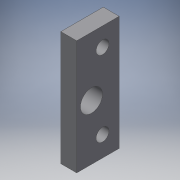
# Autodesk Inventor part: TrayPanelL
Saved by Autodesk Inventor 2017 (Build 210142000, 142)
## iProperties
Created: 2019-06-29
Part Number: TrayPanelL
Material: Generic
Document SubType Name: Modeling
Designer: DDeGo
Density: 1 g/cm^3
Appearance: Default
Author: DDeGo
Autodesk Inventor part; units mm, degrees
ref_plane "YZ Plane" through (0, 0, 0) normal (1, 0, 0) x (0, 1, 0)
ref_plane "XZ Plane" through (0, 0, 0) normal (0, 1, 0) x (-1, 0, 0)
ref_plane "XY Plane" through (0, 0, 0) normal (0, 0, 1) x (1, 0, 0)
sketch "Sketch1" plane through (0, 0, 0) normal (1, 0, 0) x (0, 1, 0)
  line L0 (0, 0) -> (11.5, 0)
  line L1 (11.5, 0) -> (11.5, 31)
  line L2 (11.5, 31) -> (0, 31)
  line L3 (0, 31) -> (0, 0)
  line L4 (0, 15) -> (4, 15) construction
  circle A0 centre (4, 15) radius 3
  line L5 (7, 26) -> (7, 5.5) construction
  circle A1 centre (7, 26) radius 1.75
  circle A2 centre (7, 5.5) radius 1.75
  dimension "d0" = 4
  dimension "d1" = 6
  dimension "d2" = 20.5
  dimension "d3" = 9.5
  dimension "d4" = 3.5
  dimension "d5" = 7
  dimension "d6" = 11.5
  dimension "d7" = 15
  dimension "d8" = 16
  constraints: 12 end point, 3 centre point, 3 coincident, 2 horizontal, 2 parallel, 1 equal radius, 1 perpendicular, 1 point on line, 1 vertical
  measures "d0" distance of L4.start L4.end
  measures "d1" diameter of A0
  measures "d2" distance of L5.start L5.end
  measures "d3" distance from line of L4 L5.end
  measures "d4" diameter of A2
  measures "d5" distance between parallel lines of L3 L5
  measures "d6" distance of L0.start L0.end
  measures "d7" distance between parallel lines of L0 L4
  measures "d8" distance between parallel lines of L4 L2
extrude "Extrusion1" add sketch "Sketch1" along normal blind 4.3
body "Solid1"
